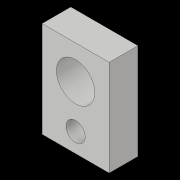
# Autodesk Inventor part: EndHole
Saved by Autodesk Inventor 2017 (Build 210142000, 142)
## iProperties
Created: 2016-12-23
Part Number: EndHole
Material: Generic
Document SubType Name: Modeling
Designer: David Kopala
Density: 1 g/cm^3
Appearance: Default
Author: David Kopala
Autodesk Inventor part; units mm, degrees
ref_plane "YZ Plane" through (0, 0, 0) normal (1, 0, 0) x (0, 1, 0)
ref_plane "XZ Plane" through (0, 0, 0) normal (0, 1, 0) x (-1, 0, 0)
ref_plane "XY Plane" through (0, 0, 0) normal (0, 0, 1) x (1, 0, 0)
sketch "Sketch1" plane through (0, 0, 0) normal (0, 0, 1) x (1, 0, 0)
  line L0 (0, 0) -> (8.89, 0)
  line L1 (8.89, 0) -> (8.89, 12.7)
  line L2 (8.89, 12.7) -> (0, 12.7)
  line L3 (0, 12.7) -> (0, 0)
  dimension "d0" = 8.89
  dimension "d1" = 12.7
  constraints: 8 end point, 2 parallel, 1 horizontal, 1 perpendicular
  measures "d0" distance of L2.end L1.end
  measures "d1" distance of L1.end L0.end
extrude "Extrusion1" add sketch "Sketch1" along normal blind 3.81
sketch "Sketch2" plane through (0, 0, 3.81) normal (0, 0, 1) x (1, 0, 0)
  circle A0 centre (4.4501, 4.445) radius 3.175
  line L0 (0, 0) -> (8.89, 0) projected
  line L1 (8.89, 0) -> (8.89, 12.7) projected
  dimension "d4" = 6.35
  dimension "d5" = 4.445
  dimension "d6" = 4.4399
  constraints: 1 centre point
  measures "d4" diameter of A0
  measures "d5" distance from line of L0 A0.centre
  measures "d6" distance from line of L1 A0.centre
hole "Hole1" at (4.4501, 4.445, 3.81) direction (0, 0, -1) diameter 5.08 depth 19.05
sketch "Sketch3" plane through (0, 0, 3.81) normal (0, 0, 1) x (1, 0, 0)
  circle A0 centre (4.445, 10.16) radius 1.27
  line L0 (8.89, 12.7) -> (0, 12.7) projected
  line L1 (8.89, 0) -> (8.89, 12.7) projected
  point P0 (0, 0)
  dimension "d14" = 2.54
  dimension "d15" = 2.54
  dimension "d16" = 4.445
  constraints: 1 centre point
  measures "d14" diameter of A0
  measures "d15" distance from line of L0 A0.centre
  measures "d16" distance from line of L1 A0.centre
extrude "Extrusion2" cut sketch "Sketch3" against normal blind 25.4
body "Solid1"
